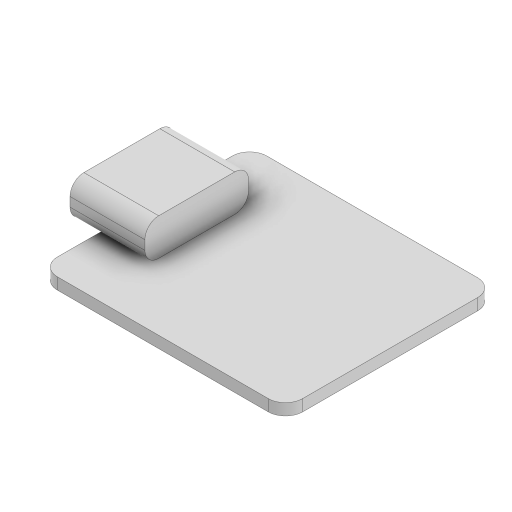
# Autodesk Inventor part: seed_arduino
Saved by Autodesk Inventor 2023 (Build 270158000, 158)
## iProperties
Created: 2023-03-26
Part Number: seed_arduino
Material: Generic
Document SubType Name: Modeling
Designer: James
Density: 1 g/cm^3
Appearance: Default
Author: James
Autodesk Inventor part; units mm, degrees
ref_plane "YZ Plane" through (0, 0, 0) normal (1, 0, 0) x (0, 1, 0)
ref_plane "XZ Plane" through (0, 0, 0) normal (0, 1, 0) x (-1, 0, 0)
ref_plane "XY Plane" through (0, 0, 0) normal (0, 0, 1) x (1, 0, 0)
sketch "Sketch1" plane through (0, 0, 0) normal (0, 1, 0) x (-1, 0, 0)
  line L0 (-9.15, 9.09) -> (9.15, 9.09)
  line L1 (10.65, 7.59) -> (10.65, -7.59)
  line L2 (9.15, -9.09) -> (-9.15, -9.09)
  line L3 (-10.65, -7.59) -> (-10.65, 7.59)
  line L4 (-10.65, 9.09) -> (10.65, -9.09) construction
  line L5 (10.65, 9.09) -> (-10.65, -9.09) construction
  arc A0 (10.65, 7.59) -> (9.15, 9.09) centre (9.15, 7.59) ccw
  arc A1 (9.15, -9.09) -> (10.65, -7.59) centre (9.15, -7.59) ccw
  arc A2 (-10.65, -7.59) -> (-9.15, -9.09) centre (-9.15, -7.59) ccw
  arc A3 (-9.15, 9.09) -> (-10.65, 7.59) centre (-9.15, 7.59) ccw
  point P0 (0, 0)
  dimension "d0" = 21.3
  dimension "d1" = 18.18
  dimension "d2" = 1.5
  constraints: 12 end point, 8 point on circle, 8 point on line, 8 tangent, 4 centre point, 3 equal radius, 2 midpoint, 2 parallel, 1 horizontal, 1 perpendicular
  measures "d0" distance of L4.end L5.end
  measures "d1" distance of L5.start L4.end
  measures "d2" radius of A0
extrude "Extrusion1" add sketch "Sketch1" along normal blind 1
sketch "Sketch2" plane through (-10.65, 0, -7.59) normal (-1, 0, 0) x (0, 0, 1)
  line L0 (4.29, 4.2) -> (10.89, 4.2)
  line L1 (12.09, 3) -> (12.09, 2.2)
  line L2 (10.89, 1) -> (4.29, 1)
  line L3 (3.09, 2.2) -> (3.09, 3)
  line L4 (3.09, 4.2) -> (12.09, 1) construction
  line L5 (12.09, 4.2) -> (3.09, 1) construction
  line L6 (0, 1) -> (15.18, 1) projected
  line L7 (0, 0) -> (15.18, 0) projected
  arc A0 (4.29, 4.2) -> (3.09, 3) centre (4.29, 3) ccw
  arc A1 (12.09, 3) -> (10.89, 4.2) centre (10.89, 3) ccw
  arc A2 (10.89, 1) -> (12.09, 2.2) centre (10.89, 2.2) ccw
  arc A3 (3.09, 2.2) -> (4.29, 1) centre (4.29, 2.2) ccw
  point P0 (7.59, 0)
  point P1 (7.59, 2.6)
  point P2 (7.59, 0)
  dimension "d5" = 9
  dimension "d6" = 3.2
  dimension "d11" = 1.2
  constraints: 12 end point, 8 point on circle, 8 point on line, 8 tangent, 4 centre point, 3 equal radius, 3 midpoint, 2 parallel, 1 collinear, 1 horizontal, 1 perpendicular, 1 vertical alignment
  measures "d5" distance of L4.end L5.end
  measures "d6" distance of L5.start L4.end
  measures "d11" radius of A0
extrude "Extrusion2" add sketch "Sketch2" along normal blind 2 and the other way blind 4.5
body "Solid1"
